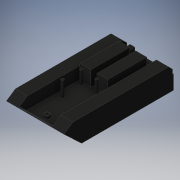
# Autodesk Inventor part: kocsi
Saved by Autodesk Inventor 2019 (Build 230136000, 136)
## iProperties
Created: 2019-02-10
Part Number: kocsi
Material: Generic
Document SubType Name: Modeling
Designer: izsoandras
Density: 1 g/cm^3
Appearance: Default
Author: izsoandras
Autodesk Inventor part; units mm, degrees
ref_plane "YZ Plane" through (0, 0, 0) normal (1, 0, 0) x (0, 1, 0)
ref_plane "XZ Plane" through (0, 0, 0) normal (0, 1, 0) x (-1, 0, 0)
ref_plane "XY Plane" through (0, 0, 0) normal (0, 0, 1) x (1, 0, 0)
sketch "Sketch1" plane through (0, 0, 0) normal (0, 1, 0) x (-1, 0, 0)
  line L0 (-45.0135, 84.3784) -> (49.9865, 84.3784)
  line L1 (49.9865, 84.3784) -> (49.9865, -94.6216)
  line L2 (49.9865, -94.6216) -> (-45.0135, -94.6216)
  line L3 (-45.0135, -94.6216) -> (-45.0135, 84.3784)
  point P0 (0, 0)
  dimension "d0" = 179
  dimension "d1" = 95
  constraints: 8 end point, 2 parallel, 1 horizontal, 1 perpendicular
  measures "d0" distance of L0.end L1.end
  measures "d1" distance of L1.end L2.end
extrude "test" add sketch "Sketch1" along normal blind 37.5
sketch "Sketch2" plane through (0, 37.5, 0) normal (0, 1, 0) x (1, 0, 0)
  line L0 (-29.9865, -83.3784) -> (25.0135, -83.3784)
  line L1 (25.0135, -83.3784) -> (25.0135, 93.6216)
  line L2 (25.0135, 93.6216) -> (-29.9865, 93.6216)
  line L3 (-29.9865, 93.6216) -> (-29.9865, -83.3784)
  line L4 (-49.9865, -84.3784) -> (45.0135, -84.3784) projected
  line L5 (-49.9865, 94.6216) -> (-49.9865, -84.3784) projected
  point P0 (0, 0)
  dimension "d4" = 55
  dimension "d5" = 177
  dimension "d6" = 1
  dimension "d7" = 20
  constraints: 8 end point, 2 parallel, 1 horizontal, 1 perpendicular
  measures "d4" distance of L0.start L0.end
  measures "d5" distance of L2.end L0.start
  measures "d6" distance between parallel lines of L4 L0
  measures "d7" distance between parallel lines of L5 L3
extrude "hasa" cut sketch "Sketch2" against normal blind 20
sketch "Sketch3" plane through (45.0135, 0, 84.3784) normal (1, 0, 0) x (0, 0, -1)
  line L0 (179, 37.5) -> (172.636, 37.5)
  line L1 (172.636, 37.5) -> (172.636, 37.5)
  line L2 (179, 31.136) -> (179, 31.136)
  line L3 (179, 31.136) -> (179, 37.5)
  line L4 (0, 37.5) -> (179, 37.5) projected
  line L5 (179, 0) -> (179, 37.5) projected
  line L6 (172.636, 37.5) -> (179, 31.136)
  point P0 (84.3784, 0)
  point P1 (172.636, 31.136)
  dimension "d10" = 6.364
  dimension "d11" = 6.364
  dimension "d12" = 0
  dimension "d13" = 0
  dimension "d14" = 6.364
  dimension "d15" = 45
  constraints: 10 end point, 2 parallel, 2 point on line, 1 horizontal, 1 perpendicular
  measures "d10" distance of point (172.636, 31.136) L2.end
  measures "d11" distance of L0.end point (172.636, 31.136)
  measures "d12" distance between parallel lines of L4 L0
  measures "d13" distance between parallel lines of L5 L3
  measures "d14" distance of L1.end point (172.636, 31.136)
  measures "d15" angle of L1 L6
extrude "hátsó levágás" cut sketch "Sketch3" against normal through all
sketch "Sketch4" plane through (45.0135, 0, -94.6216) normal (0, 0, -1) x (-1, 0, 0)
  line L0 (95, 0) -> (95, 37.5) projected
  line L1 (0, 0) -> (95, 0)
  line L2 (95, 0) -> (95, 23.136)
  line L3 (95, 23.136) -> (0, 23.136)
  line L4 (0, 23.136) -> (0, 0)
  line L5 (95, 31.136) -> (0, 31.136) projected
  point P0 (45.0135, 0)
  dimension "d18" = 8
  constraints: 8 end point, 2 parallel, 1 horizontal, 1 perpendicular, 1 point on line
  measures "d18" distance between parallel lines of L5 L3
extrude "hátsó kiszögellés" add sketch "Sketch4" along normal blind 2
sketch "Sketch6" plane through (45.0135, 31.136, -94.6216) normal (0, 0, -1) x (-1, 0, 0)
  line L0 (20, 1) -> (20, -13.636) projected
  line L1 (95, -8) -> (0, -8) projected
  line L2 (20, 1) -> (75, 1)
  line L3 (75, 1) -> (75, -8)
  line L4 (75, -8) -> (20, -8)
  line L5 (20, -8) -> (20, 1)
  line L6 (75, 1) -> (75, 6.364) projected
  line L7 (20, 1) -> (75, 1) projected
  point P0 (45.0135, -31.136)
  dimension "d21" = 0
  constraints: 8 end point, 2 parallel, 2 point on line, 1 collinear, 1 horizontal, 1 perpendicular
  measures "d21" distance between parallel lines of L7 L2
extrude "Extrusion5" cut sketch "Sketch6" against normal up to surface (1 mm away)
sketch "Sketch7" plane through (0, 17.5, 0) normal (0, 1, 0) x (1, 0, 0)
  line L0 (25.0135, 93.6216) -> (-29.9865, 93.6216) projected
  line L1 (-23.9865, 93.6216) -> (-15.9865, 93.6216)
  line L2 (-15.9865, 93.6216) -> (-15.9865, 79.6216)
  line L3 (-15.9865, 79.6216) -> (-23.9865, 79.6216)
  line L4 (-23.9865, 79.6216) -> (-23.9865, 93.6216)
  line L5 (-29.9865, -83.3784) -> (-29.9865, 88.2577) projected
  point P0 (0, 0)
  dimension "d24" = 14
  dimension "d25" = 8
  dimension "d26" = 6
  constraints: 8 end point, 2 parallel, 1 horizontal, 1 perpendicular, 1 point on line
  measures "d24" distance of L1.end L2.end
  measures "d25" distance of L2.end L3.end
  measures "d26" distance between parallel lines of L4 L5
extrude "táp csati" add sketch "Sketch7" along normal blind 15
sketch "Sketch8" plane through (45.0135, 0, 84.3784) normal (1, 0, 0) x (0, 0, -1)
  line L0 (0, 0) -> (0, 37.5) projected
  line L1 (0, 37.5) -> (15, 37.5)
  line L2 (15, 37.5) -> (15, 37.5)
  line L3 (0, 27.5) -> (0, 27.5)
  line L4 (0, 27.5) -> (0, 37.5)
  line L5 (15, 37.5) -> (0, 27.5)
  point P0 (84.3784, 0)
  point P1 (15, 27.5)
  dimension "d29" = 10
  dimension "d30" = 10
  dimension "d31" = 15
  dimension "d32" = 15
  constraints: 10 end point, 2 parallel, 2 point on line, 1 horizontal, 1 perpendicular
  measures "d29" distance of L1.end point (15, 27.5)
  measures "d30" distance of L2.end point (15, 27.5)
  measures "d31" distance of L3.start point (15, 27.5)
  measures "d32" distance of L0.end L1.end
extrude "első levágás" cut sketch "Sketch8" against normal through all
sketch "Sketch9" plane through (0, 17.5, 0) normal (0, 1, 0) x (1, 0, 0)
  line L0 (-27.9865, 79.1216) -> (-9.9865, 79.1216)
  line L1 (-9.9865, 79.1216) -> (-9.9865, 15.1216)
  line L2 (-9.9865, 15.1216) -> (-27.9865, 15.1216)
  line L3 (-27.9865, 15.1216) -> (-27.9865, 79.1216)
  line L4 (-29.9865, -69.3784) -> (-29.9865, 88.2577) projected
  line L5 (25.0135, 93.6216) -> (-15.9865, 93.6216) projected
  line L6 (25.0135, 88.2577) -> (25.0135, -69.3784) projected
  point P0 (0, 0)
  dimension "d35" = 64
  dimension "d36" = 18
  dimension "d37" = 2
  dimension "d38" = 14.5
  constraints: 8 end point, 2 parallel, 1 horizontal, 1 perpendicular
  measures "d35" distance of L0.end L1.end
  measures "d36" distance of L1.end L2.end
  measures "d37" distance between parallel lines of L4 L3
  measures "d38" distance between parallel lines of L5 L0
extrude "motor jobb" add sketch "Sketch9" along normal blind 25
sketch "Sketch10" plane through (0, 17.5, 0) normal (0, 1, 0) x (1, 0, 0)
  line L0 (0.0135, 79.1216) -> (18.0135, 79.1216)
  line L1 (18.0135, 79.1216) -> (18.0135, 15.1216)
  line L2 (18.0135, 15.1216) -> (0.0135, 15.1216)
  line L3 (0.0135, 15.1216) -> (0.0135, 79.1216)
  line L4 (25.0135, 88.2577) -> (25.0135, -69.3784) projected
  line L5 (25.0135, 93.6216) -> (-15.9865, 93.6216) projected
  point P0 (0, 0)
  dimension "d45" = 7
  dimension "d46" = 18
  dimension "d47" = 64
  dimension "d48" = 14.5
  constraints: 8 end point, 2 parallel, 1 horizontal, 1 perpendicular
  measures "d45" distance between parallel lines of L4 L1
  measures "d46" distance between parallel lines of L3 L1
  measures "d47" distance of L2.end L0.start
  measures "d48" distance between parallel lines of L5 L0
extrude "motor bal" add sketch "Sketch10" along normal blind 25
sketch "Sketch11" plane through (45.0135, 0, -96.6216) normal (1, 0, 0) x (0, 0, -1)
  line L0 (-181, 0) -> (-181, 27.5) projected
  line L1 (-181, 27.5) -> (-151.8278, 0)
  line L2 (0, 0) -> (-181, 0) projected
  line L3 (-166, 37.5) -> (-181, 27.5) projected
  point P0 (-96.6216, 0)
  dimension "d51" = 77
  constraints: 2 end point, 1 point on line
  measures "d51" angle of L3 L1
extrude "eleje alső levágás" cut sketch "Sketch11" against normal through all
sketch "Sketch12" plane through (-29.9865, 23.136, -94.6216) normal (1, 0, 0) x (0, 0, -1)
  line L0 (-168.3919, -5.636) -> (-1, -5.636) projected
  line L1 (-178, 3.4213) -> (-168.3919, -5.636) projected
  line L2 (-168.3919, -5.636) -> (-178, 3.4213)
  line L3 (-178, 3.4213) -> (-176.7937, 4.7009)
  line L4 (-176.7937, 4.7009) -> (-165.8282, -5.636)
  line L5 (-167.1856, -4.3564) -> (-168.3919, -5.636)
  line L6 (-164, 14.364) -> (-178, 5.0306) projected
  line L7 (-176.7937, 4.7009) -> (-178, 5.0306)
  line L8 (-178, 5.0306) -> (-178, 3.4213)
  line L9 (-168.3919, -5.636) -> (-165.8282, -5.636)
  point P0 (-94.6216, -23.136)
  constraints: 14 end point, 2 parallel, 2 perpendicular, 2 point on line, 1 collinear, 1 vertical
extrude "eleje korrekció" add sketch "Sketch12" along normal up to next
sketch "Sketch13" plane through (0, 17.5, 0) normal (0, 1, 0) x (1, 0, 0)
  circle A0 centre (-18.7965, -22.8984) radius 2.3
  line L0 (-29.9865, -69.3784) -> (-29.9865, 88.2577) projected
  line L1 (-29.9865, -83.3784) -> (25.0135, -83.3784) projected
  line L2 (45.0135, -84.3784) -> (-49.9865, -84.3784) projected
  point P0 (0, 0)
  dimension "d56" = 4.6
  dimension "d57" = 11.19
  dimension "d74" = 61.48
  constraints: 1 centre point
  measures "d56" diameter of A0
  measures "d57" distance from line of L0 A0.centre
  measures "d74" distance from line of L2 A0.centre
extrude "oszlop1" add sketch "Sketch13" along normal blind 26.01
sketch "Sketch14" plane through (0, 17.5, 0) normal (0, 1, 0) x (1, 0, 0)
  circle A0 centre (-21.6865, 10.8216) radius 2.3
  line L0 (-29.9865, -69.3784) -> (-29.9865, 88.2577) projected
  line L1 (-27.9865, 15.1216) -> (-9.9865, 15.1216) projected
  point P0 (0, 0)
  dimension "d61" = 4.6
  dimension "d70" = 8.3
  dimension "d71" = 4.3
  constraints: 1 centre point
  measures "d61" diameter of A0
  measures "d70" distance from line of L0 A0.centre
  measures "d71" distance from line of L1 A0.centre
extrude "oszlop2" add sketch "Sketch14" along normal blind 22.3
sketch "Sketch15" plane through (0, 17.5, 0) normal (0, 1, 0) x (1, 0, 0)
  circle A0 centre (4.6685, 9.7966) radius 2.205
  line L0 (45.0135, -84.3784) -> (-49.9865, -84.3784) projected
  line L1 (25.0135, 88.2577) -> (25.0135, -69.3784) projected
  point P0 (0, 0)
  dimension "d64" = 4.41
  dimension "d72" = 94.175
  dimension "d73" = 20.345
  constraints: 1 centre point
  measures "d64" diameter of A0
  measures "d72" distance from line of L0 A0.centre
  measures "d73" distance from line of L1 A0.centre
extrude "oszlop3" add sketch "Sketch15" along normal blind 22.2
sketch "Sketch16" plane through (0, 17.5, 0) normal (0, 1, 0) x (1, 0, 0)
  circle A0 centre (15.4235, -54.5484) radius 2.35
  line L0 (45.0135, -84.3784) -> (-49.9865, -84.3784) projected
  line L1 (25.0135, 88.2577) -> (25.0135, -69.3784) projected
  point P0 (0, 0)
  dimension "d67" = 4.7
  dimension "d75" = 29.83
  dimension "d76" = 9.59
  constraints: 1 centre point
  measures "d67" diameter of A0
  measures "d75" distance from line of L0 A0.centre
  measures "d76" distance from line of L1 A0.centre
extrude "oszlop4" add sketch "Sketch16" along normal blind 10.12
sketch "Sketch17" plane through (0, 17.5, 0) normal (0, 1, 0) x (1, 0, 0)
  circle A0 centre (-1.9556, -65.0384) radius 4
  line L0 (45.0135, -84.3784) -> (-49.9865, -84.3784) projected
  point P0 (0, 0)
  dimension "d77" = 8
  dimension "d78" = 19.34
  constraints: 1 centre point
  measures "d77" diameter of A0
  measures "d78" distance from line of L0 A0.centre
extrude "Extrusion16" add sketch "Sketch17" along normal blind 6.11
sketch "Sketch18" plane through (-1.9556, 23.61, 65.0384) normal (0, 1, 0) x (1, 0, 0)
  circle A0 centre (0, 0) radius 2.6
  circle A1 centre (0, 0) radius 4 projected
  point P0 (1.9556, 65.0384)
  dimension "d81" = 1.4
  constraints: 1 centre point
  measures "d81" radial gap between concentric circles of A0 A1
extrude "Extrusion17" cut sketch "Sketch18" against normal blind 4.6 contours A0
sketch "Sketch19" plane through (-1.9556, 19.01, 65.0384) normal (0, 1, 0) x (1, 0, 0)
  circle A0 centre (0, 0) radius 1.5
  point P0 (1.9556, 65.0384)
  dimension "d84" = 3
  constraints: 1 centre point
  measures "d84" diameter of A0
extrude "Extrusion18" cut sketch "Sketch19" against normal through all
sketch "Sketch20" plane through (0, 17.5, 0) normal (0, 1, 0) x (1, 0, 0)
  circle A0 centre (-2.7865, 80.7416) radius 4
  line L0 (-49.9865, 96.6216) -> (45.0135, 96.6216) projected
  line L1 (25.0135, 88.2577) -> (25.0135, -69.3784) projected
  point P0 (0, 0)
  dimension "d87" = 8
  dimension "d88" = 15.88
  dimension "d89" = 27.8
  constraints: 1 centre point
  measures "d87" diameter of A0
  measures "d88" distance from line of L0 A0.centre
  measures "d89" distance from line of L1 A0.centre
extrude "Extrusion19" add sketch "Sketch20" along normal blind 7.5
sketch "Sketch21" plane through (0, 25, 0) normal (0, 1, 0) x (1, 0, 0)
  circle A0 centre (-2.7865, 80.7416) radius 2.58
  arc A1 (0.8708, 79.1216) -> (0.0135, 77.8851) centre (-2.7865, 80.7416) ccw projected
  point P0 (0, 0)
  dimension "d92" = 0
  dimension "d93" = 0
  dimension "d94" = 1.42
  constraints: 1 centre point
  measures "d92" distance of A1.centre A0.centre
  measures "d93" distance of A1.centre A0.centre
  measures "d94" radial gap between concentric circles of A1 A0
extrude "Extrusion20" cut sketch "Sketch21" against normal blind 4.92
sketch "Sketch22" plane through (-2.7865, 20.08, -80.7416) normal (0, 1, 0) x (1, 0, 0)
  circle A0 centre (0, 0) radius 2
  point P0 (2.7865, -80.7416)
  dimension "d97" = 4
  constraints: 1 centre point
  measures "d97" diameter of A0
extrude "Extrusion21" cut sketch "Sketch22" against normal through all
equation "\"d11\" = d10"
equation "\"d14\" = d10"
body "Solid1"
